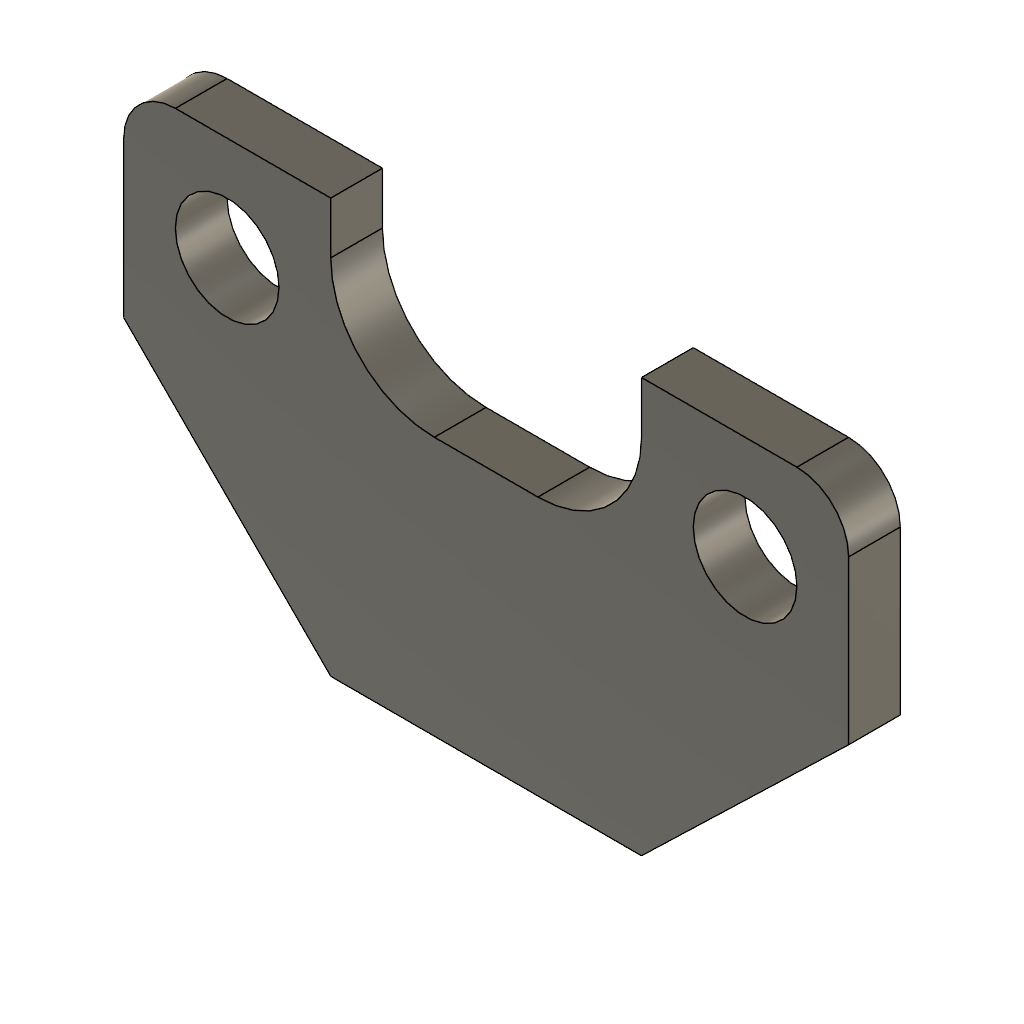
exercise 13 (Autodesk Fusion 360 design; units mm, degrees)
part number: 2026-10-07-17-22-23-943
Autodesk Fusion 360 part; units mm, degrees
sketch "Sketch1" plane through (0, 0, 0) normal (0, 1, 0) x (1, 0, 0)
  circle A0 centre (-40.1897, -10) radius 5
  circle A1 centre (9.8103, -10) radius 5
  line L0 (-50.1897, 0) -> (-50.1897, -15)
  line L1 (-45.1897, -20) -> (-30.1897, -20)
  line L2 (-30.1897, -20) -> (-30.1897, -15)
  line L3 (-20.1897, -5) -> (-10.1897, -5)
  line L4 (-0.1897, -15) -> (-0.1897, -20)
  line L5 (-0.1897, -20) -> (14.8103, -20)
  line L6 (19.8103, -15) -> (19.8103, 0.7211)
  line L7 (19.8103, 0.7211) -> (-0.1897, 20)
  line L8 (-0.1897, 20) -> (-30.1897, 20)
  line L9 (-30.1897, 20) -> (-50.1897, 0)
  arc A2 (-50.1897, -15) -> (-45.1897, -20) centre (-45.1897, -15) ccw
  arc A3 (14.8103, -20) -> (19.8103, -15) centre (14.8103, -15) ccw
  arc A4 (-20.1897, -5) -> (-30.1897, -15) centre (-20.1897, -15) ccw
  arc A5 (-0.1897, -15) -> (-10.1897, -5) centre (-10.1897, -15) ccw
  point P0 (-50.1897, -20)
  point P1 (-30.1897, -5)
  point P2 (-0.1897, -5)
  dimension "d1" = 10
  dimension "d2" = 10
  dimension "d3" = 50
  dimension "d4" = 70
  dimension "d5" = 20
  dimension "d6" = 30
  dimension "d7" = 30
  dimension "d8" = 20
  dimension "d9" = 10
  dimension "d10" = 20
  dimension "d11" = 30
  dimension "d12" = 40
  dimension "d13" = 15
  dimension "d14" = 5
  dimension "d15" = 5
  dimension "d16" = 10
  dimension "d17" = 10
  constraint vertical L0
  constraint perpendicular L0 L1
  constraint perpendicular L1 L2
  constraint perpendicular L2 L3
  constraint perpendicular L3 L4
  constraint perpendicular L4 L5
  constraint perpendicular L3 L6
  constraint perpendicular L6 L8
  constraint coincident P0 L0
  constraint coincident P0 L1
  constraint tangent L0 A2
  constraint tangent L1 A2
  constraint tangent L5 A3
  constraint tangent L6 A3
  constraint coincident P1 L2
  constraint coincident P1 L3
  constraint tangent L2 A4
  constraint tangent L3 A4
  constraint coincident P2 L3
  constraint coincident P2 L4
  constraint tangent L3 A5
  constraint tangent L4 A5
  measures "d1" diameter of A0
  measures "d2" diameter of A1
  measures "d3" distance of A0.centre A1.centre
  measures "d4" horizontal distance of L0.start L6.end
  measures "d5" horizontal distance of L0.start L8.end
  measures "d6" distance of L7.end L8.end
  measures "d7" distance of P1 P2
  measures "d8" distance of P0 L1.end
  measures "d9" horizontal distance of A0.centre P0
  measures "d10" vertical distance of L0.start L8.end
  measures "d11" vertical distance of A0.centre L8.end
  measures "d12" vertical distance of P0 L8.end
  measures "d13" distance of P2 L4.end
  measures "d14" radius of A2
  measures "d15" radius of A3
  measures "d16" radius of A4
  measures "d17" radius of A5
extrude "Extrude1" add sketch "Sketch1" along normal blind 5
